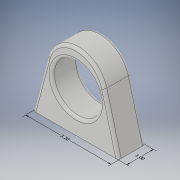
# Autodesk Inventor part: CapStone Handle
Saved by Autodesk Inventor 2018 (Build 220112000, 112)
## iProperties
Created: 2020-01-09
Part Number: CapStone Handle
Material: Generic
Document SubType Name: Modeling
Designer: AOFUser
Density: 1 g/cm^3
Appearance: Default
Author: AOFUser
Autodesk Inventor part; units mm, degrees
ref_plane "YZ Plane" through (0, 0, 0) normal (1, 0, 0) x (0, 1, 0)
ref_plane "XZ Plane" through (0, 0, 0) normal (0, 1, 0) x (-1, 0, 0)
ref_plane "XY Plane" through (0, 0, 0) normal (0, 0, 1) x (1, 0, 0)
sketch "Sketch2" plane through (0, 0, 0) normal (0, 1, 0) x (-1, 0, 0)
  line L0 (0, 0) -> (-81.28, 0)
  line L1 (-81.28, 0) -> (-81.28, -25.4)
  line L2 (-81.28, -25.4) -> (0, -25.4)
  line L3 (0, -25.4) -> (0, 0)
  dimension "d2" = 81.28
  dimension "d3" = 25.4
  constraints: 8 end point, 2 parallel, 1 horizontal, 1 perpendicular
  measures "d2" distance of L2.end L1.end
  measures "d3" distance of L1.end L0.end
extrude "Extrusion1" add sketch "Sketch2" along normal blind 76.2
sketch "Sketch3" plane through (81.28, 0, -25.4) normal (0, 0, -1) x (-1, 0, 0)
  line L0 (81.28, 76.2) -> (0, 76.2) projected
  line L1 (40.64, 76.2) -> (40.64, 0)
  line L2 (0, 0) -> (0, 76.2) projected
  line L3 (0, 38.1) -> (81.28, 38.1)
  line L4 (81.28, 0) -> (81.28, 76.2) projected
  circle A0 centre (40.64, 38.1) radius 22.86
  dimension "d6" = 45.72
  constraints: 4 end point, 4 midpoint, 1 centre point, 1 vertical
  measures "d6" diameter of A0
extrude "Extrusion2" cut sketch "Sketch3" against normal blind 25.4 contours A0 L3 L1 | L1 L3 A0 | A0 L1 L3 | L1 A0 L3
chamfer "Chamfer1" distance 20.32 distance2 76.2 1 edges at (81.28, 76.2, -12.7) measured on face at (54.1867, 76.2, -8.4667)
chamfer "Chamfer2" distance 20.32 distance2 76.2 1 edges at (0, 76.2, -12.7) measured on face at (40.6403, 76.2, -16.9333)
fillet "Fillet1" radius 27.94 2 edges at (60.9605, 76.2, -12.7) (20.3195, 76.2, -12.7)
fillet "Fillet2" radius 2.54 8 edges at (63.5, 38.1, 0) (63.5, 38.1, -25.4) (74.4578, 25.5841, 0) (6.8222, 25.5841, 0) (40.64, 71.9079, 0) (6.8222, 25.5841, -25.4) (74.4578, 25.5841, -25.4) (40.64, 71.9079, -25.4)
sketch "Sketch5" plane through (0, 0, 0) normal (0, -1, 0) x (1, 0, 0)
  line L0 (2.6288, 0) -> (78.6512, 0) projected
  line L1 (40.64, 0) -> (40.64, -25.4)
  line L2 (78.6512, -25.4) -> (2.6288, -25.4) projected
  line L3 (0, -12.7) -> (81.4991, -12.7)
  line L4 (40.7495, -12.7) -> (51.1635, -12.7)
  line L5 (51.1635, -12.7) -> (51.1635, -6.604)
  line L6 (51.1635, -6.604) -> (30.3355, -6.604)
  line L7 (30.3355, -6.604) -> (30.3355, -18.796)
  line L8 (30.3355, -18.796) -> (51.1635, -18.796)
  line L9 (51.1635, -18.796) -> (51.1635, -12.7)
  point P0 (0, 0)
  dimension "d23" = 10.414
  dimension "d24" = 6.096
  dimension "d25" = 20.828
  dimension "d26" = 12.192
  constraints: 16 end point, 4 perpendicular, 3 midpoint, 2 horizontal, 1 point on line
  measures "d23" distance of L4.start L4.end
  measures "d24" distance of L4.end L5.end
  measures "d25" distance of L5.end L6.end
  measures "d26" distance of L6.end L7.end
extrude "Extrusion4" cut sketch "Sketch5" against normal blind 5.08
body "Solid1"
